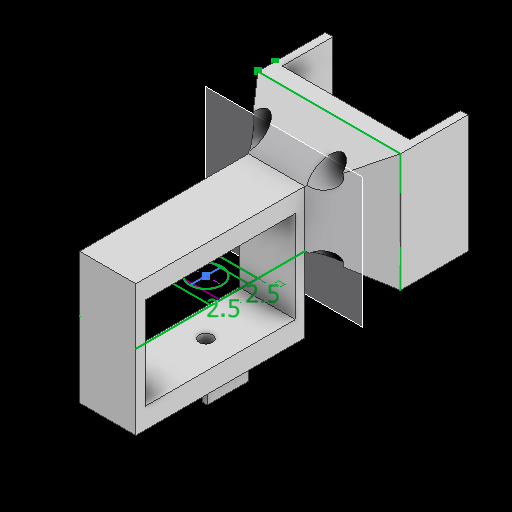
# Autodesk Inventor part: spring_connector
Saved by Autodesk Inventor 2025.1 (Build 291241000, 241)
## iProperties
Created: 2024-08-22
Part Number: spring_connector
Material: 일반
Document SubType Name: Modeling
Designer: ojs08
Density: 1 g/cm^3
Appearance: 기본값
Author: ojs08
Autodesk Inventor part; units mm, degrees
ref_plane "YZ Plane" through (0, 0, 0) normal (1, 0, 0) x (0, 1, 0)
ref_plane "XZ Plane" through (0, 0, 0) normal (0, 1, 0) x (-1, 0, 0)
ref_plane "XY Plane" through (0, 0, 0) normal (0, 0, 1) x (1, 0, 0)
sketch "스케치1" plane through (0, 0, 0) normal (0, 0, 1) x (1, 0, 0)
  line L0 (0, 0) -> (38, 0)
  line L1 (38, 0) -> (38, -31.5)
  line L2 (38, -31.5) -> (0, -31.5)
  line L3 (0, -31.5) -> (0, 0)
  dimension "d0" = 38
  dimension "d1" = 31.5
  constraints: 8 end point, 2 parallel, 1 coincident, 1 horizontal, 1 perpendicular
  measures "d0" distance of L1.end L2.end
  measures "d1" distance of L0.end L1.end
extrude "돌출1" add sketch "스케치1" along normal blind 18
sketch "스케치2" plane through (0, 0, 0) normal (0, 0, -1) x (-1, 0, 0)
  line L0 (0, -31.5) -> (-38, -31.5) projected
  line L1 (0, 0) -> (0, -31.5) projected
  line L2 (-38, 0) -> (0, 0) projected
  line L3 (-38, -31.5) -> (-38, 0) projected
  line L4 (-2, -31.5) -> (-2, 0)
  line L5 (0, -31.5) -> (-38, -31.5) projected
  line L6 (-36, -31.5) -> (-36, 0)
  dimension "d4" = 2
  dimension "d5" = 2
  constraints: 4 end point, 4 point on line, 2 perpendicular
  measures "d4" distance between parallel lines of L1 L4
  measures "d5" distance between parallel lines of L3 L6
extrude "돌출2" cut sketch "스케치2" against normal blind 13.5 contours L0 L6 L2 L4
sketch "스케치3" plane through (0, 0, 18) normal (0, 0, 1) x (1, 0, 0)
  point P0 (0, 0)
ref_plane "작업 평면1" through (0, 0, 30) normal (0, 0, 1) x (1, 0, 0)
sketch "스케치4" plane through (0, 0, 18) normal (0, 0, 1) x (1, 0, 0)
  line L0 (0, -31.5) -> (38, -31.5) projected
  line L1 (38, -31.5) -> (38, 0) projected
  line L2 (38, 0) -> (0, 0) projected
  line L3 (0, 0) -> (0, -31.5) projected
sketch "스케치5" plane through (0, 0, 30) normal (0, 0, 1) x (1, 0, 0)
  line L0 (0, 0) -> (0, -31.5) projected
  line L1 (0, -31.5) -> (38, -31.5) projected
  line L2 (9.5, -8.25) -> (24.5, -8.25)
  line L3 (24.5, -8.25) -> (24.5, -23.25)
  line L4 (24.5, -23.25) -> (9.5, -23.25)
  line L5 (9.5, -23.25) -> (9.5, -8.25)
  point P0 (17, -15.75)
  point P1 (17, -23.25)
  dimension "d9" = 17
  dimension "d10" = 15.75
  dimension "d11" = 15
  dimension "d12" = 15
  dimension "d13" = 7.5
  dimension "d14" = 7.5
  constraints: 8 end point, 2 parallel, 1 horizontal, 1 midpoint, 1 perpendicular
  measures "d9" distance from line of L0 point (17, -15.75)
  measures "d10" distance from line of L1 point (17, -15.75)
  measures "d11" distance of L2.start L2.end
  measures "d12" distance of L2.end L3.end
  measures "d13" distance from line of L3 point (17, -15.75)
  measures "d14" distance of point (17, -23.25) point (17, -15.75)
loft "로프트1" add profiles "스케치5" section 2 edges at (19, -31.5, 18) (38, -15.75, 18) (19, 0, 18) (0, -15.75, 18)
sketch "스케치6" plane through (0, 0, 13.5) normal (0, 0, -1) x (-1, 0, 0)
  line L0 (-2, -31.5) -> (-36, -31.5) projected
  line L1 (-2, 0) -> (-2, -31.5) projected
  line L2 (-36, 0) -> (-2, 0) projected
  line L3 (-36, -31.5) -> (-36, 0) projected
  circle A0 centre (-7, -26) radius 2
  circle A1 centre (-7, -6) radius 2
  circle A2 centre (-27, -26) radius 2
  circle A3 centre (-27, -6) radius 2
  point P0 (0, 0)
  dimension "d19" = 4
  dimension "d20" = 5
  dimension "d21" = 5.5
  dimension "d24" = 20
  dimension "d31" = 20
  constraints: 4 centre point, 1 horizontal, 1 vertical, 6 other
  measures "d19" diameter of A0
  measures "d20" distance from line of L1 A0.centre
  measures "d21" distance from line of L0 A0.centre
  measures "d24" distance of A0.centre A1.centre
  measures "d31" distance of A0.centre A2.centre
extrude "돌출3" cut sketch "스케치6" against normal blind 2 contours A0 | A1 | A2 | A3
sketch "스케치7" plane through (0, 0, 13.5) normal (0, 0, -1) x (-1, 0, 0)
  circle A0 centre (-7, -26) radius 2 projected
  circle A1 centre (-7, -6) radius 2 projected
  circle A2 centre (-27, -6) radius 2 projected
  circle A3 centre (-27, -26) radius 2 projected
  circle A4 centre (-7, -26) radius 2.7017
  point P0 (0, 0)
  constraints: 1 centre point
ref_plane "작업 평면2" through (0, 0, 15.5) normal (0, 0, -1) x (-1, 0, 0)
sketch "스케치8" plane through (0, 0, 13.5) normal (0, 0, -1) x (-1, 0, 0)
  circle A0 centre (-7, -26) radius 2.7017 projected
  circle A1 centre (-7, -26) radius 2 projected
  circle A2 centre (-7, -26) radius 3
  point P0 (0, 0)
  dimension "d39" = 0.7017
  dimension "d40" = 6
  constraints: 1 centre point, 1 concentric
  measures "d39" radial gap between concentric circles of A0 A1
  measures "d40" diameter of A2
sketch "스케치9" plane through (0, 0, 13.5) normal (0, 0, -1) x (-1, 0, 0)
  circle A0 centre (-7, -6) radius 3
  circle A1 centre (-27, -6) radius 3
  circle A2 centre (-27, -26) radius 3
  circle A3 centre (-27, -26) radius 2 projected
  circle A4 centre (-27, -6) radius 2 projected
  circle A5 centre (-7, -6) radius 2 projected
  point P0 (0, 0)
  dimension "d41" = 6
  dimension "d42" = 6
  dimension "d43" = 6
  constraints: 3 centre point, 3 concentric
  measures "d41" diameter of A0
  measures "d42" diameter of A1
  measures "d43" diameter of A2
sketch "스케치10" plane through (0, 0, 13.5) normal (0, 0, -1) x (-1, 0, 0)
  circle A0 centre (-7, -26) radius 3 projected
  circle A1 centre (-27, -26) radius 3 projected
  circle A2 centre (-27, -6) radius 3 projected
  circle A3 centre (-7, -6) radius 3 projected
  point P0 (0, 0)
extrude "돌출4" cut sketch "스케치8" against normal blind 16 from surface at -2 contours A0 | A1 | A2
extrude "돌출5" cut sketch "스케치9" against normal blind 16 from surface at -2 contours A2 | A3
extrude "돌출6" cut sketch "스케치10" against normal blind 16 from surface at -2 contours A3
sketch "스케치11" plane through (0, 0, 13.5) normal (0, 0, -1) x (-1, 0, 0)
  circle A0 centre (-27, -6) radius 3
  circle A1 centre (-27, -6) radius 2 projected
  point P0 (0, 0)
  dimension "d50" = 6
  constraints: 1 centre point, 1 concentric
  measures "d50" diameter of A0
extrude "돌출7" cut sketch "스케치11" against normal blind 16 from surface at -2 contours A0 | A1
sketch "스케치12" plane through (0, 0, 30) normal (0, 0, 1) x (1, 0, 0)
  line L0 (9.5, -23.25) -> (9.5, -8.25) projected
  line L1 (24.5, -23.25) -> (9.5, -23.25) projected
  line L2 (24.5, -8.25) -> (24.5, -23.25) projected
  line L3 (9.5, -8.25) -> (24.5, -8.25) projected
  point P0 (0, 0)
extrude "돌출8" add sketch "스케치12" along normal blind 25
sketch "스케치14" plane through (9.5, -23.25, 30) normal (0, -1, 0) x (1, 0, 0)
  circle A0 centre (7.5, 18.85) radius 4.25 projected
  circle A1 centre (7.5, 18.85) radius 4.25 projected
  line L0 (7.5, 23.1) -> (7.5, 14.6)
  circle A2 centre (7.5, 18.85) radius 4.25 projected
  point P0 (-9.5, -30)
  constraints: 2 end point, 1 point on circle, 1 vertical, 1 vertical alignment, 1 other
sketch "스케치15" plane through (9.5, -23.25, 30) normal (0, -1, 0) x (1, 0, 0)
  line L0 (15, 0) -> (0, 0) projected
  line L1 (15, 0) -> (15, 25) projected
  line L2 (0, 25) -> (15, 25) projected
  line L3 (0, 0) -> (0, 25) projected
  line L4 (15, 22.5) -> (0, 22.5)
  line L5 (15, 15) -> (0, 15)
  line L6 (15, 12.5) -> (0, 12.5)
  point P0 (-9.5, -30)
  dimension "d60" = 2.5
  dimension "d61" = 2.5
  constraints: 6 end point, 4 point on line, 2 midpoint, 2 perpendicular
  measures "d60" distance between parallel lines of L2 L4
  measures "d61" distance between parallel lines of L5 L6
sketch "스케치16" plane through (0, 0, 55) normal (0, 0, 1) x (1, 0, 0)
  line L0 (24.5, -23.25) -> (24.5, -8.25) projected
  line L1 (24.5, -8.25) -> (9.5, -8.25) projected
  line L2 (9.5, -8.25) -> (9.5, -23.25) projected
  line L3 (9.5, -23.25) -> (24.5, -23.25) projected
  point P0 (0, 0)
extrude "돌출10" add sketch "스케치16" along normal blind 20
sketch "스케치17" plane through (9.5, -23.25, 30) normal (0, -1, 0) x (1, 0, 0)
  line L0 (15, 0) -> (0, 0) projected
  line L1 (15, 0) -> (15, 45) projected
  line L2 (0, 45) -> (15, 45) projected
  line L3 (0, 0) -> (0, 45) projected
  line L4 (15, 0) -> (15, 45) projected
  line L5 (15, 42.5) -> (0, 42.5)
  point P0 (-9.5, -30)
  dimension "d64" = 2.5
  constraints: 2 end point, 2 point on line, 1 perpendicular
  measures "d64" distance between parallel lines of L2 L5
sketch "스케치18" plane through (9.5, -23.25, 30) normal (0, -1, 0) x (1, 0, 0)
  line L0 (15, 12.5) -> (0, 12.5) projected
  line L1 (15, 15) -> (0, 15) projected
  line L2 (15, 0) -> (15, 45) projected
  line L3 (0, 0) -> (0, 45) projected
  point P0 (-9.5, -30)
sketch "스케치19" plane through (9.5, -23.25, 30) normal (0, -1, 0) x (1, 0, 0)
  line L0 (15, 0) -> (15, 45) projected
  line L1 (15, 15.0424) -> (15, 12.8959)
  line L2 (15, 12.5) -> (0, 12.5) projected
  line L3 (15, 12.5) -> (15, 15.0424)
  line L4 (0, 12.5) -> (0, 15.0424)
  line L5 (0, 0) -> (0, 45) projected
  point P0 (-9.5, -30)
  constraints: 6 end point, 3 point on line, 1 vertical
sketch "스케치20" plane through (9.5, -23.25, 30) normal (0, -1, 0) x (1, 0, 0)
  line L0 (15, 0) -> (15, 45) projected
  line L1 (15, 2.5) -> (0, 2.5)
  line L2 (0, 0) -> (0, 45) projected
  line L3 (15, 0) -> (0, 0) projected
  point P0 (-9.5, -30)
  dimension "d65" = 2.5
  constraints: 2 end point, 2 point on line, 1 horizontal
  measures "d65" distance between parallel lines of L3 L1
extrude "돌출11" add sketch "스케치20" along normal blind 20
extrude "돌출12" add sketch "스케치17" along normal blind 20 contours L5 L3 L2 L1
sketch "스케치21" plane through (9.5, -23.25, 32.5) normal (0, 0, 1) x (1, 0, 0)
  line L0 (0, 0) -> (15, 0) projected
  line L1 (0, 0) -> (0, -20) projected
  line L2 (15, -20) -> (0, -20) projected
  line L3 (15, 0) -> (15, -20) projected
  line L4 (15, 0) -> (15, -20) projected
  line L5 (15, -18.5) -> (0, -18.5)
  point P0 (-9.5, 23.25)
  point P1 (15, -18.5)
  dimension "d70" = 1.5
  constraints: 2 end point, 2 point on line, 1 perpendicular
  measures "d70" distance between parallel lines of L5 L2
extrude "돌출13" add sketch "스케치21" along normal up to surface (40 mm away) contours L5 L3 L2 L1
sketch "스케치22" plane through (9.5, -23.25, 32.5) normal (0, -1, 0) x (1, 0, 0)
  circle A0 centre (7.5, 16.35) radius 4.25 projected
  point P0 (-9.5, -32.5)
sketch "스케치23" plane through (9.5, -43.25, 30) normal (0, -1, 0) x (1, 0, 0)
  circle A0 centre (7.5, 18.85) radius 4.25 projected
  circle A1 centre (7.5, 18.85) radius 1.75
  point P0 (-9.5, -30)
  dimension "d73" = 3.5
  constraints: 1 centre point, 1 coincident
  measures "d73" diameter of A1
extrude "돌출14" cut sketch "스케치23" against normal up to surface (1.5 mm away) contours A1
sketch "스케치24" plane through (9.5, -43.25, 30) normal (0, -1, 0) x (1, 0, 0)
  line L0 (12.5, 23.5) -> (11.25, 23.5)
  line L1 (11.25, 23.5) -> (11.25, 12.5)
  line L2 (11.25, 12.5) -> (12.5, 12.5)
  line L3 (12.5, 12.5) -> (12.5, 23.5)
  line L4 (3.75, 23.5) -> (2.5, 23.5)
  line L5 (2.5, 23.5) -> (2.5, 12.5)
  line L6 (2.5, 12.5) -> (3.75, 12.5)
  line L7 (3.75, 12.5) -> (3.75, 23.5)
  circle A0 centre (7.5, 18.85) radius 1.75 projected
  line L8 (0, 0) -> (15, 0) projected
  line L9 (15, 0) -> (15, 45) projected
  line L10 (0, 45) -> (0, 0) projected
  point P0 (-9.5, -30)
  dimension "d76" = 3.75
  dimension "d77" = 3.75
  dimension "d78" = 12.5
  dimension "d79" = 12.5
  dimension "d80" = 11
  dimension "d81" = 11
  dimension "d82" = 2.5
  dimension "d83" = 2.5
  constraints: 16 end point, 4 parallel, 2 horizontal, 2 perpendicular
  measures "d76" distance from line of L1 A0.centre
  measures "d77" distance from line of L7 A0.centre
  measures "d78" distance between parallel lines of L8 L2
  measures "d79" distance between parallel lines of L8 L6
  measures "d80" distance of L2.end L0.start
  measures "d81" distance of L4.end L5.end
  measures "d82" distance between parallel lines of L9 L3
  measures "d83" distance between parallel lines of L5 L10
extrude "돌출15" add sketch "스케치24" along normal blind 5 contours L3 L2 L1 L0 | L7 L6 L5 L4
sketch "스케치25" plane through (9.5, -8.25, 30) normal (-1, 0, 0) x (0, 0, 1)
  line L0 (2.5, -15) -> (42.5, -15) projected
  line L1 (45, -35) -> (0, -35) projected
  line L2 (45, 0) -> (45, -35) projected
  line L3 (0, 0) -> (45, 0) projected
  line L4 (0, -15) -> (0, 0) projected
  line L5 (0, -15) -> (0, -35) projected
  line L6 (2.5, -33.5) -> (42.5, -33.5) projected
  line L7 (2.5, -15) -> (2.5, -33.5) projected
  line L8 (2.5, -15) -> (42.5, -15) projected
  line L9 (42.5, -15) -> (42.5, -33.5) projected
  line L10 (2.5, -15) -> (42.5, -15)
  line L11 (42.5, -15) -> (42.5, -5)
  line L12 (42.5, -5) -> (2.5, -5)
  line L13 (2.5, -5) -> (2.5, -15)
  point P0 (-30, 8.25)
  dimension "d86" = 5
  constraints: 8 end point, 2 parallel, 1 horizontal, 1 perpendicular
  measures "d86" distance between parallel lines of L3 L12
extrude "돌출16" cut sketch "스케치25" against normal up to surface (15 mm away) contours L13 L12 L11 L0
sketch "스케치26" plane through (9.5, -8.25, 30) normal (-1, 0, 0) x (0, 0, 1)
  line L0 (2.5, -33.5) -> (2.5, -5) projected
  line L1 (2.5, -5) -> (42.5, -5) projected
  line L2 (42.5, -5) -> (42.5, -33.5) projected
  line L3 (2.5, -33.5) -> (42.5, -33.5) projected
  line L4 (45, -35) -> (0, -35) projected
  line L5 (45, 0) -> (45, -35) projected
  line L6 (0, 0) -> (45, 0) projected
  line L7 (0, -15) -> (0, 0) projected
  line L8 (0, -15) -> (0, -35) projected
  line L9 (2.5, -29.5) -> (42.5, -29.5)
  point P0 (-30, 8.25)
  dimension "d89" = 4
  constraints: 2 end point, 2 point on line, 1 perpendicular
  measures "d89" distance between parallel lines of L9 L3
extrude "돌출17" add sketch "스케치26" against normal up to surface (15 mm away) contours L0 L9 L2 L3
sketch "스케치27" plane through (9.5, -43.25, 30) normal (0, -1, 0) x (1, 0, 0)
  circle A0 centre (7.5, 18.85) radius 1.75 projected
  point P0 (-9.5, -30)
sketch "스케치28" plane through (17, -41.75, 48.85) normal (0, -1, 0) x (1, 0, 0)
  circle A0 centre (0, 0) radius 1.75 projected
  point P0 (-17, -48.85)
extrude "돌출18" cut sketch "스케치28" against normal up to surface (4 mm away)
